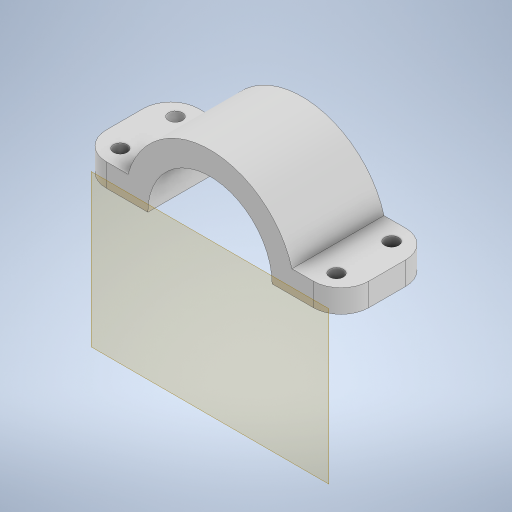
# Autodesk Inventor part: Capa suporte
Saved by Autodesk Inventor 2024.1 (Build 281209000, 209)
## iProperties
Created: 2024-11-08
Part Number: Capa suporte
Material: Genérico
Document SubType Name: Modeling
Designer: dimit
Density: 1 g/cm^3
Appearance: Padrão
Author: dimit
Autodesk Inventor part; units mm, degrees
ref_plane "YZ Plane" through (0, 0, 0) normal (1, 0, 0) x (0, 1, 0)
ref_plane "XZ Plane" through (0, 0, 0) normal (0, 1, 0) x (-1, 0, 0)
ref_plane "XY Plane" through (0, 0, 0) normal (0, 0, 1) x (1, 0, 0)
ref_plane "Plano de trabalho1" through (0, 0, 0) normal (0, 0, 1) x (1, 0, 0)
sketch "Esboço1" plane through (0, 0, 0) normal (0, 0, 1) x (1, 0, 0)
  arc A0 (-40.8144, 85.0081) -> (-13.8144, 85.0195) centre (-27.3144, 85.0138) ccw
  circle A1 centre (-27.3144, 85.0138) radius 13.5
  line L0 (-40.8144, 85.0081) -> (-45.8144, 85.006)
  line L1 (-45.8144, 85.006) -> (-55.8144, 85.0017)
  line L2 (-55.8144, 85.0017) -> (-13.8144, 85.0195)
  line L3 (-13.8144, 85.0195) -> (-8.8144, 85.0216)
  line L4 (-8.8144, 85.0216) -> (1.1856, 85.0259)
  line L5 (1.1856, 85.0259) -> (1.1834, 90.0259)
  line L6 (1.1834, 90.0259) -> (-14.7766, 90.0191)
  line L7 (-55.8144, 85.0017) -> (-55.8166, 90.0017)
  line L8 (-55.8166, 90.0017) -> (-39.8565, 90.0085)
  line L9 (-27.3144, 98.5138) -> (-27.3166, 103.5138)
  arc A2 (-8.8144, 85.0216) -> (-45.8144, 85.006) centre (-27.3144, 85.0138) ccw
  point P0 (0, 0)
  point P1 (-40.8144, 85.0081)
  point P2 (-13.8144, 85.0195)
  point P3 (-9.5051, 90.0213)
  point P4 (-45.1281, 90.0062)
  dimension "d0" = 27
  dimension "d1" = 13.5
  dimension "d2" = 5
  dimension "d3" = 10
  dimension "d4" = 5
  dimension "d5" = 10
  dimension "d6" = 5
  dimension "d7" = 5
  dimension "d8" = 5
  constraints: 20 end point, 8 point on circle, 4 perpendicular, 3 centre point, 3 point on line, 1 coincident, 1 collinear, 1 concentric
  measures "d0" distance of L0.start L2.end
  measures "d1" radius of A0
  measures "d2" distance of L0.start L0.end
  measures "d3" distance of L0.end L1.end
  measures "d4" distance of L2.end L3.end
  measures "d5" distance of L3.end L4.end
  measures "d6" distance of L4.end L5.end
  measures "d7" distance of L1.end L7.end
  measures "d8" distance of L9.start L9.end
extrude "Extrusão1" add sketch "Esboço1" against normal blind 20 contours L0 A2 L8 A1 | L8 A2 L9 A1 | L1 L7 L8 A2 | A1 L6 A2 L3 | L9 A2 L6 A1 | A2 L6 L5 L4
fillet "Arredondamento1" radius 6 4 edges at (1.1845, 87.5259, 0) (1.1845, 87.5259, -20) (-55.8155, 87.5017, 0) (-55.8155, 87.5017, -20)
sketch "Esboço2" plane through (-13.8144, 85.0195, -20) normal (0.0004, -1, 0) x (1, 0.0004, 0)
  arc A0 (9.2495, 14.6999) -> (10.7509, 14.6999) centre (10.0003, 16.0018) ccw
  circle A1 centre (10.0003, 16.0018) radius 1.5029
  arc A2 (9.2495, 2.6941) -> (10.7509, 2.6875) centre (10.0061, 4.0358) ccw
  circle A3 centre (10.0061, 4.0358) radius 1.5402
  arc A4 (-37.7345, 14.6999) -> (-36.2329, 14.6999) centre (-36.9837, 16.0022) ccw
  circle A5 centre (-36.9837, 16.0022) radius 1.5032
  line L0 (-36.2329, 2.6941) -> (-37.7345, 2.6941)
  line L1 (-37.7345, 2.6941) -> (-36.2546, 4.1926)
  arc A6 (-37.7345, 2.6941) -> (-36.2329, 2.6941) centre (-36.9837, 4.0136) ccw
  circle A7 centre (-36.9837, 4.0136) radius 1.5181
  point P0 (13.7784, 20)
  point P1 (10.7509, 2.6875)
  point P2 (9.2495, 2.6941)
  point P3 (10.7509, 14.6999)
  point P4 (9.2495, 14.6999)
  point P5 (-36.2329, 14.6999)
  point P6 (-37.7345, 14.6999)
  point P7 (-37.7345, 2.6941)
  point P8 (-36.2329, 2.6941)
  constraints: 8 centre point, 8 point on circle, 4 coincident, 4 end point, 3 concentric, 1 horizontal
extrude "Extrusão2" cut sketch "Esboço2" against normal blind 20
